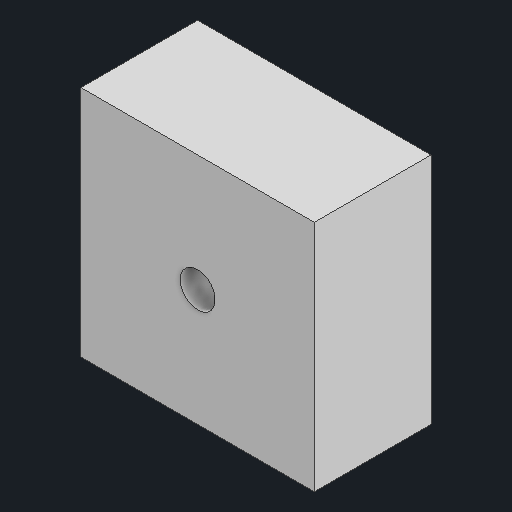
# Autodesk Inventor part: 26_hole_countersink
Saved by Autodesk Inventor 2027 (Build 310192060, 192F)
## iProperties
Created: 2026-07-12
Part Number: 26_hole_countersink
Material: Generic
Document SubType Name: Modeling
Designer: vmiguel
Density: 1 g/cm^3
Appearance: Default
Author: vmiguel
Autodesk Inventor part; units mm, degrees
ref_plane "YZ Plane" through (0, 0, 0) normal (1, 0, 0) x (0, 1, 0)
ref_plane "XZ Plane" through (0, 0, 0) normal (0, 1, 0) x (-1, 0, 0)
ref_plane "XY Plane" through (0, 0, 0) normal (0, 0, 1) x (1, 0, 0)
sketch "Sketch1" plane through (0, 0, 0) normal (0, 0, 1) x (1, 0, 0)
  line L0 (0, 0) -> (40, 0)
  line L1 (40, 0) -> (40, 40)
  line L2 (40, 40) -> (0, 40)
  line L3 (0, 40) -> (0, 0)
  constraints: 8 end point, 2 parallel, 1 horizontal, 1 perpendicular
extrude "Extrusion1" add sketch "Sketch1" along normal blind 20
sketch "Sketch2" plane through (0, 0, 0) normal (0, 0, 1) x (1, 0, 0)
  point P0 (20, 20)
hole "Hole1" at (20, 20, 0) direction (0, 0, 1) diameter 6 end through all countersink diameter 14 countersink angle 90
body "Solid1"
